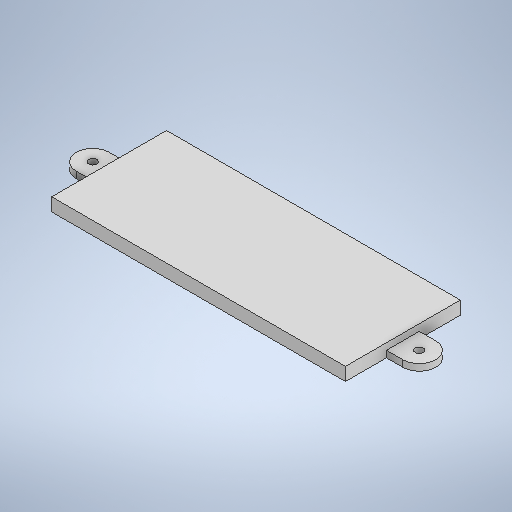
# Autodesk Inventor part: Fuslage cover
Saved by Autodesk Inventor 2025.3 (Build 293356030, 356C)
## iProperties
Created: 2025-08-23
Part Number: Fuslage cover
Material: Generic
Document SubType Name: Modeling
Designer: mateo
Density: 1 g/cm^3
Appearance: Default
Author: mateo
Autodesk Inventor part; units mm, degrees
ref_plane "YZ Plane" through (0, 0, 0) normal (1, 0, 0) x (0, 1, 0)
ref_plane "XZ Plane" through (0, 0, 0) normal (0, 1, 0) x (-1, 0, 0)
ref_plane "XY Plane" through (0, 0, 0) normal (0, 0, 1) x (1, 0, 0)
sketch "Sketch1" plane through (0, 0, 0) normal (0, 1, 0) x (-1, 0, 0)
  line L0 (19, 96) -> (-160, 96)
  line L1 (-160, 96) -> (-160, 26)
  line L2 (-160, 26) -> (19, 26)
  line L3 (19, 26) -> (19, 96)
  point P0 (0, 0)
  dimension "d0" = 179
  dimension "d1" = 70
  constraints: 8 end point, 2 parallel, 1 horizontal, 1 perpendicular
  measures "d0" distance of L0.start L0.end
  measures "d1" distance of L0.end L1.end
extrude "Extrusion1" add sketch "Sketch1" along normal blind 8
sketch "Sketch2" plane through (0, 8, 0) normal (0, 1, 0) x (1, 0, 0)
  circle A0 centre (-29, -61) radius 10
  line L0 (-29, -71) -> (-14.7125, -71)
  line L1 (-29, -51) -> (-14.2875, -51)
  line L2 (-14.7125, -71) -> (-14.2875, -51)
  line L3 (160, -26) -> (-19, -26) projected
  line L4 (70.5, -26) -> (70.5, -114.3)
  circle A1 centre (170, -61) radius 10
  line L5 (170, -71) -> (155.7125, -71)
  line L6 (170, -51) -> (155.2875, -51)
  line L7 (155.7125, -71) -> (155.2875, -51)
  line L8 (-19, -96) -> (160, -96) projected
  line L9 (-19, -26) -> (-19, -96) projected
  point P0 (0, 0)
  point P1 (-19, -61)
  dimension "d5" = 20
  dimension "d14" = 25
  dimension "d16" = 10
  constraints: 14 end point, 5 symmetric about line, 4 point on circle, 2 centre point, 2 horizontal, 2 midpoint, 2 tangent, 1 vertical, 1 other
  measures "d5" diameter of A0
  measures "d14" distance between parallel lines of L1 L3
  measures "d16" distance of point (-19, -61) A0.centre
extrude "Extrusion2" add sketch "Sketch2" against normal blind 8 contours A0 | L9 L0 A0 | A0 L1 L9 | L9 L1 L2 L0 | A1 | A1 L5 L7 L6
sketch "Sketch3" plane through (0, 8, 0) normal (0, 1, 0) x (1, 0, 0)
  arc A0 (-29, -51) -> (-29, -71) centre (-29, -61) ccw projected
  circle A1 centre (-29, -61) radius 2.5
  arc A2 (170, -71) -> (170, -51) centre (170, -61) ccw projected
  circle A3 centre (170, -61) radius 2.5
  point P0 (0, 0)
  dimension "d8" = 5
  dimension "d9" = 5
  constraints: 2 centre point, 2 coincident
  measures "d8" diameter of A1
  measures "d9" diameter of A3
extrude "Extrusion3" cut sketch "Sketch3" against normal blind 8
sketch "Sketch4" plane through (0, 8, 0) normal (0, 1, 0) x (1, 0, 0)
  line L0 (-19, -26) -> (-19, -96) projected
  line L1 (-19, -41.275) -> (-45.0875, -41.275)
  line L2 (-45.0875, -41.275) -> (-45.0875, -80.9625)
  line L3 (-45.0875, -80.9625) -> (-19, -80.9625)
  line L4 (-19, -80.9625) -> (-19, -41.275)
  line L5 (160, -96) -> (160, -26) projected
  line L6 (160, -41.275) -> (180.975, -41.275)
  line L7 (180.975, -41.275) -> (180.975, -82.55)
  line L8 (180.975, -82.55) -> (160, -82.55)
  line L9 (160, -82.55) -> (160, -41.275)
  point P0 (0, 0)
  point P1 (-19, -51)
  point P2 (160, -51)
  point P3 (160, -82.55)
  point P4 (-19, -80.9625)
  constraints: 16 end point, 4 parallel, 2 horizontal, 2 perpendicular, 2 point on line
extrude "Extrusion4" cut sketch "Sketch4" against normal blind 4
body "Solid1"
